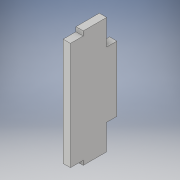
# Autodesk Inventor part: battlebotspinner20mmplate
Saved by Autodesk Inventor 2019 (Build 230136000, 136)
## iProperties
Created: 2018-08-13
Part Number: battlebotspinner20mmplate
Material: Generic
Document SubType Name: Modeling
Designer: Kitte_X
Density: 1 g/cm^3
Appearance: Default
Author: Kitte_X
Autodesk Inventor part; units mm, degrees
ref_plane "YZ Plane" through (0, 0, 0) normal (1, 0, 0) x (0, 1, 0)
ref_plane "XZ Plane" through (0, 0, 0) normal (0, 1, 0) x (-1, 0, 0)
ref_plane "XY Plane" through (0, 0, 0) normal (0, 0, 1) x (1, 0, 0)
sketch "Sketch1" plane through (0, 0, 0) normal (1, 0, 0) x (0, 1, 0)
  line L0 (159, 32) -> (159, -32)
  line L1 (159, -32) -> (89, -32)
  line L2 (89, -32) -> (89, -60)
  line L3 (89, -60) -> (-89, -60)
  line L4 (159, 32) -> (147, 32)
  line L5 (147, 32) -> (147, 67)
  line L6 (147, 67) -> (-147, 67)
  line L7 (-147, 67) -> (-147, 32)
  line L8 (-147, 32) -> (-159, 32)
  line L9 (-159, 32) -> (-159, -32)
  line L10 (-159, -32) -> (-89, -32)
  line L11 (-89, -32) -> (-89, -60)
  point P0 (0, 0)
  point P1 (159, 0)
  point P2 (0, 67)
  dimension "d0" = 64
  dimension "d1" = 70
  dimension "d2" = 178
  dimension "d3" = 28
  dimension "d4" = 12
  dimension "d5" = 35
  dimension "d6" = 12
  dimension "d7" = 64
  dimension "d8" = 70
  dimension "d9" = 35
  constraints: 24 end point, 9 perpendicular, 2 horizontal, 2 midpoint, 1 horizontal alignment, 1 vertical, 1 vertical alignment
  measures "d0" distance of L0.start L0.end
  measures "d1" distance of L0.end L1.end
  measures "d2" distance of L2.end L3.end
  measures "d3" distance of L1.end L2.end
  measures "d4" distance of L0.start L4.end
  measures "d5" distance of L4.end L5.end
  measures "d6" distance of L7.end L8.end
  measures "d7" distance of L8.end L9.end
  measures "d8" distance of L9.end L10.end
  measures "d9" distance of L6.end L7.end
extrude "Extrusion1" add sketch "Sketch1" along normal blind 20
body "Solid1"
